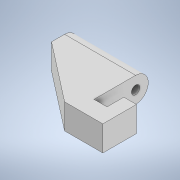
# Autodesk Inventor part: Pi3B_spacer_R
Saved by Autodesk Inventor 2022 (Build 260153000, 153)
## iProperties
Created: 2023-01-27
Part Number: Pi3B_spacer_R
Material: Generic
Document SubType Name: Modeling
Designer: scott
Density: 1 g/cm^3
Appearance: Default
Author: scott
Autodesk Inventor part; units mm, degrees
ref_plane "YZ Plane" through (0, 0, 0) normal (1, 0, 0) x (0, 1, 0)
ref_plane "XZ Plane" through (0, 0, 0) normal (0, 1, 0) x (-1, 0, 0)
ref_plane "XY Plane" through (0, 0, 0) normal (0, 0, 1) x (1, 0, 0)
sketch "Sketch1" plane through (0, 0, 0) normal (0, 1, 0) x (-1, 0, 0)
  line L0 (0, 0) -> (23, 0)
  line L1 (23, 0) -> (23, 17)
  line L2 (23, 17) -> (0, 17)
  line L3 (0, 17) -> (0, 0)
  line L4 (6.1, 13) -> (3, 13)
  line L5 (3, 13) -> (3, 0)
  line L6 (3, 0) -> (6.1, 0)
  line L7 (6.1, 0) -> (6.1, 13)
  line L8 (23, 17) -> (9.1, 17)
  line L9 (9.1, 17) -> (9.1, 0)
  line L10 (9.1, 0) -> (23, 0)
  line L11 (23, 0) -> (23, 17)
  line L12 (9.1, 17) -> (23, 6.2)
  point P0 (9.1, 17)
  dimension "d0" = 23
  dimension "d1" = 17
  dimension "d2" = 3.1
  dimension "d3" = 3
  dimension "d4" = 3
  dimension "d5" = 6.2
  dimension "d17" = 13
  constraints: 26 end point, 6 parallel, 3 horizontal, 3 perpendicular, 3 point on line
  measures "d0" distance of L2.end L1.end
  measures "d1" distance of L1.end L0.end
  measures "d2" distance between parallel lines of L5 L7
  measures "d3" distance between parallel lines of L3 L5
  measures "d4" distance between parallel lines of L7 L9
  measures "d5" distance from line of L0 L12.end
  measures "d17" distance between parallel lines of L0 L4
extrude "Extrusion1" add sketch "Sketch1" along normal blind 6 contours L3 L2 L9 L0 L7 L4 L5 | L12 L1 L0 L9
sketch "Sketch2" plane through (-23, 0, 0) normal (-1, 0, 0) x (0, 0, 1)
  circle A0 centre (3.1, 3) radius 3
  line L0 (0, 0) -> (13, 0) projected
  line L1 (0, 0) -> (0, 6) projected
  line L2 (17, 6) -> (0, 6) projected
  line L3 (0, 0) -> (6.2302, 0)
  line L4 (6.2302, 0) -> (6.2302, 6)
  line L5 (6.2302, 6) -> (0, 6)
  line L6 (0, 6) -> (0, 0)
  circle A1 centre (3.1, 3) radius 1
  point P0 (3.1, 6)
  point P1 (3.1, 0)
  dimension "d8" = 3.1
  dimension "d9" = 2
  constraints: 8 end point, 2 centre point, 2 parallel, 1 coincident, 1 horizontal, 1 perpendicular, 1 point on line, 1 tangent
  measures "d8" distance from line of L1 A0.centre
  measures "d9" diameter of A1
extrude "Extrusion2" cut sketch "Sketch2" against normal up to surface (20 mm away) contours A0 L0 L1 L2 | A1
sketch "Sketch3" plane through (0, 6, 0) normal (0, 1, 0) x (1, 0, 0)
  line L0 (-3, 0) -> (-3, -13) projected
  line L1 (0, 0) -> (-3, 0) projected
  line L2 (-3, -9) -> (0, -9)
  line L3 (0, -9) -> (0, 0)
  line L4 (0, 0) -> (-3, 0)
  line L5 (-3, 0) -> (-3, -9)
  line L6 (-3, -13) -> (-6.1, -13) projected
  line L7 (-9.1, -17) -> (0, -17) projected
  dimension "d13" = 8
  constraints: 8 end point, 2 parallel, 1 horizontal, 1 perpendicular, 1 point on line
  measures "d13" distance between parallel lines of L7 L2
extrude "Extrusion3" cut sketch "Sketch3" against normal blind 10
body "Solid1"
